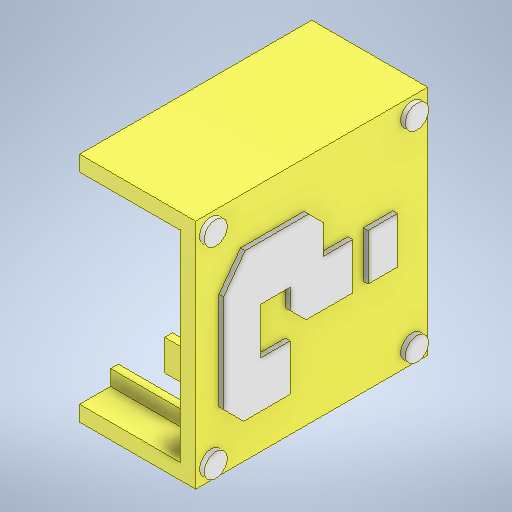
# Autodesk Inventor part: vraagblok2
Saved by Autodesk Inventor 2025 (Build 290162000, 162)
## iProperties
Created: 2024-05-27
Part Number: vraagblok2
Material: Generic
Document SubType Name: Modeling
Designer: wardv
Density: 1 g/cm^3
Appearance: Smooth - Yellow
Author: wardv
Autodesk Inventor part; units mm, degrees
ref_plane "YZ Plane" through (0, 0, 0) normal (1, 0, 0) x (0, 1, 0)
ref_plane "XZ Plane" through (0, 0, 0) normal (0, 1, 0) x (-1, 0, 0)
ref_plane "XY Plane" through (0, 0, 0) normal (0, 0, 1) x (1, 0, 0)
sketch "Sketch1" plane through (0, 0, 0) normal (0, 0, 1) x (1, 0, 0)
  line L0 (0, 0) -> (75, 0)
  line L1 (75, 0) -> (75, 150)
  line L2 (75, 150) -> (0, 150)
  line L3 (0, 150) -> (0, 0)
  dimension "d0" = 75
  dimension "d1" = 150
  constraints: 8 end point, 2 parallel, 1 horizontal, 1 perpendicular
  measures "d0" distance of L2.end L1.end
  measures "d1" distance between parallel lines of L0 L2
extrude "Extrusion1" add sketch "Sketch1" along normal blind 10
sketch "Sketch2" plane through (0, 0, 10) normal (0, 0, 1) x (1, 0, 0)
  line L0 (48, 85) -> (53, 85)
  line L1 (53, 85) -> (53, 19)
  line L2 (53, 19) -> (48, 19)
  line L3 (48, 19) -> (48, 14)
  line L4 (48, 14) -> (58, 14)
  line L5 (58, 14) -> (58, 90)
  line L6 (58, 90) -> (48, 90)
  line L7 (75, 150) -> (0, 150) projected
  line L8 (0, 150) -> (0, 0) projected
  line L9 (48, 85) -> (48, 90)
  dimension "d4" = 10
  dimension "d5" = 76
  dimension "d6" = 66
  dimension "d8" = 60
  dimension "d9" = 5
  dimension "d10" = 10
  dimension "d11" = 53
  dimension "d12" = 5
  dimension "d13" = 5
  constraints: 16 end point, 6 perpendicular, 1 horizontal
  measures "d4" distance of L5.end L6.end
  measures "d5" distance of L4.end L5.end
  measures "d6" distance of L0.end L1.end
  measures "d8" distance between parallel lines of L7 L6
  measures "d9" distance between parallel lines of L5 L1
  measures "d10" distance of L3.end L4.end
  measures "d11" distance between parallel lines of L8 L1
  measures "d12" distance of L2.end L3.end
  measures "d13" distance of L0.start L0.end
extrude "Extrusion2" add sketch "Sketch2" along normal blind 5
sketch "Sketch3" plane through (53, 19, 10) normal (-1, 0, 0) x (0, 0, 1)
  line L0 (5, 66) -> (5, 0) projected
  line L1 (5, 66) -> (3, 66)
  line L2 (3, 66) -> (3, 56)
  line L3 (3, 56) -> (5, 56)
  line L4 (5, 56) -> (5, 66)
  line L5 (5, 0) -> (5, -5) projected
  line L6 (5, 0) -> (3, 0)
  line L7 (3, 0) -> (3, 10)
  line L8 (3, 10) -> (5, 10)
  line L9 (5, 10) -> (5, 0)
  point P0 (-10, -19)
  point P1 (5, 10)
  point P2 (5, 56)
  dimension "d16" = 2
  dimension "d17" = 10
  dimension "d18" = 10
  dimension "d19" = 2
  constraints: 16 end point, 4 parallel, 2 horizontal, 2 perpendicular
  measures "d16" distance of L3.end L2.end
  measures "d17" distance of L1.end L2.end
  measures "d18" distance of L6.end L7.end
  measures "d19" distance between parallel lines of L0 L7
extrude "Extrusion3" add sketch "Sketch3" along normal blind 3
sketch "Sketch4" plane through (0, 0, 10) normal (0, 0, 1) x (1, 0, 0)
  line L0 (0, 150) -> (0, 0) projected
  line L1 (0, 10) -> (65, 10)
  line L2 (65, 10) -> (65, 140)
  line L3 (65, 140) -> (0, 140)
  line L4 (75, 150) -> (0, 150) projected
  line L5 (75, 0) -> (75, 150) projected
  line L6 (0, 0) -> (75, 0) projected
  point P0 (0, 140)
  dimension "d22" = 10
  dimension "d24" = 10
  dimension "d25" = 10
  constraints: 6 end point, 3 perpendicular, 1 point on line
  measures "d22" distance between parallel lines of L4 L3
  measures "d24" distance between parallel lines of L5 L2
  measures "d25" distance between parallel lines of L6 L1
extrude "Extrusion4" add sketch "Sketch4" along normal blind 140 contours L4 L5 L6 L0 L1 L2 L3
sketch "Sketch5" plane through (0, 10, 10) normal (0, 1, 0) x (1, 0, 0)
  line L0 (0, 10) -> (0, -140) projected
  line L1 (0, -115) -> (50, -115)
  line L2 (50, -115) -> (50, -85)
  line L3 (50, -85) -> (0, -85)
  line L4 (0, -115) -> (0, -120)
  line L5 (0, -120) -> (55, -120)
  line L6 (55, -120) -> (55, -80)
  line L7 (55, -80) -> (0, -80)
  line L8 (0, -85) -> (0, -80)
  line L9 (0, -140) -> (75, -140) projected
  dimension "d28" = 50
  dimension "d29" = 30
  dimension "d30" = 5
  dimension "d31" = 55
  dimension "d32" = 40
  dimension "d37" = 20
  constraints: 16 end point, 5 perpendicular, 4 point on line, 1 horizontal, 1 parallel
  measures "d28" distance of L1.start L1.end
  measures "d29" distance of L1.end L2.end
  measures "d30" distance of L1.start L4.end
  measures "d31" distance of L4.end L5.end
  measures "d32" distance of L5.end L6.end
  measures "d37" distance between parallel lines of L9 L5
extrude "Extrusion5" add sketch "Sketch5" along normal blind 10 contours L7 L6 L5 L0 L1 L2 L3
sketch "Sketch6" plane through (0, 10, 95) normal (0, 1, 0) x (1, 0, 0)
  line L0 (50, -30) -> (50, 0) projected
  line L1 (0, 0) -> (0, -30) projected
  line L2 (50, -30) -> (0, -30)
  line L3 (0, -30) -> (0, 0)
  line L4 (0, 0) -> (50, 0)
  line L5 (50, 0) -> (50, -30)
  point P0 (0, 95)
  point P1 (0, -30)
  constraints: 8 end point, 2 parallel, 1 horizontal, 1 perpendicular
extrude "Extrusion6" cut sketch "Sketch6" against normal blind 10
sketch "Sketch7" plane through (50, 0, 125) normal (-1, 0, 0) x (0, 0, 1)
  line L0 (-30, 0) -> (-30, 20) projected
  line L1 (0, 20) -> (0, 0) projected
  line L2 (-30, 20) -> (0, 20)
  line L3 (0, 20) -> (0, 17)
  line L4 (0, 17) -> (-30, 17)
  line L5 (-30, 17) -> (-30, 20)
  line L6 (0, 10) -> (-30, 10)
  line L7 (-30, 10) -> (-30, 13)
  line L8 (-30, 13) -> (0, 13)
  line L9 (0, 13) -> (0, 10)
  point P0 (-125, 0)
  point P1 (0, 13)
  point P2 (-30, 13)
  point P3 (0, 20)
  dimension "d38" = 3
  dimension "d39" = 3
  constraints: 16 end point, 4 parallel, 2 horizontal, 2 perpendicular, 2 point on line, 1 midpoint
  measures "d38" distance between parallel lines of L6 L8
  measures "d39" distance between parallel lines of L2 L4
extrude "Extrusion7" add sketch "Sketch7" along normal blind 5 contours L0 L8 L1 L6 | L0 L2 L1 L4
sketch "Sketch8" plane through (0, 0, 0) normal (-1, 0, 0) x (0, 0, 1)
  circle A0 centre (5, 120) radius 2.5
  circle A1 centre (5, 30) radius 2.5
  circle A2 centre (60, 5) radius 2.5
  circle A3 centre (120, 145) radius 2.5
  circle A4 centre (30, 145) radius 2.5
  line L0 (0, 0) -> (95, 0) projected
  line L1 (0, 150) -> (0, 0) projected
  line L2 (0, 150) -> (150, 150) projected
  line L3 (10, 140) -> (150, 140) projected
  line L4 (150, 150) -> (150, 140) projected
  dimension "d42" = 5
  dimension "d43" = 5
  dimension "d44" = 5
  dimension "d45" = 5
  dimension "d46" = 5
  dimension "d47" = 5
  dimension "d48" = 60
  dimension "d49" = 5
  dimension "d50" = 30
  dimension "d51" = 5
  dimension "d52" = 30
  dimension "d53" = 30
  dimension "d54" = 5
  dimension "d55" = 5
  dimension "d56" = 30
  constraints: 5 centre point
  measures "d42" diameter of A0
  measures "d43" diameter of A1
  measures "d44" diameter of A2
  measures "d45" diameter of A3
  measures "d46" diameter of A4
  measures "d47" distance from line of L0 A2.centre
  measures "d48" distance from line of L1 A2.centre
  measures "d49" distance from line of L1 A1.centre
  measures "d50" distance from line of L0 A1.centre
  measures "d51" distance from line of L1 A0.centre
  measures "d52" distance from line of L2 A0.centre
  measures "d53" distance from line of L1 A4.centre
  measures "d54" distance from line of L2 A4.centre
  measures "d55" distance from line of L3 A3.centre
  measures "d56" distance from line of L4 A3.centre
extrude "Extrusion8" cut sketch "Sketch8" against normal blind 5
sketch "Sketch9" plane through (75, 0, 0) normal (1, 0, 0) x (0, 0, -1)
  line L0 (-92, 25.5) -> (-92, 55.5)
  line L1 (-92, 55.5) -> (-111, 55.5)
  line L2 (-111, 55.5) -> (-111, 85.5)
  line L3 (-111, 85.5) -> (-92, 85.5)
  line L4 (-92, 85.5) -> (-92, 72.5)
  line L5 (-92, 72.5) -> (-81.582, 62.082)
  line L6 (-81.582, 62.082) -> (-51.582, 62.082)
  line L7 (-51.582, 62.082) -> (-51.582, 92.082)
  line L8 (-51.582, 92.082) -> (-70.582, 92.082)
  line L9 (-70.582, 92.082) -> (-70.582, 111.082)
  line L10 (-70.582, 111.082) -> (-80, 120.5)
  line L11 (-80, 120.5) -> (-121, 120.5)
  line L12 (-135, 38.5) -> (-122, 25.5)
  line L13 (-122, 25.5) -> (-92, 25.5)
  line L14 (-41.582, 62.082) -> (-22.582, 62.082)
  line L15 (-22.582, 62.082) -> (-22.582, 92.082)
  line L16 (-22.582, 92.082) -> (-41.582, 92.082)
  line L17 (-41.582, 92.082) -> (-41.582, 62.082)
  line L18 (-150, 0) -> (-150, 150) projected
  line L19 (0, 150) -> (-150, 150) projected
  line L20 (-135, 38.5) -> (-135, 101.5)
  line L21 (-135, 101.5) -> (-121, 120.5)
  line L22 (-10, 10) -> (-150, 10) projected
  circle A0 centre (-140, 10) radius 7.5
  line L23 (-10, 140) -> (-150, 140) projected
  circle A1 centre (-140, 140) radius 7.5
  line L24 (-10, 10) -> (-90, 10) projected
  circle A2 centre (-10, 10) radius 7.5
  line L25 (-10, 140) -> (-10, 10) projected
  circle A3 centre (-10, 140) radius 7.5
  line L26 (0, 0) -> (0, 150) projected
  point P0 (-100.5, 120.5)
  point P1 (-51.582, 77.082)
  point P2 (-135, 70)
  dimension "d59" = 30
  dimension "d60" = 19
  dimension "d61" = 30
  dimension "d62" = 19
  dimension "d63" = 13
  dimension "d64" = 30
  dimension "d65" = 30
  dimension "d66" = 19
  dimension "d67" = 19
  dimension "d68" = 41
  dimension "d69" = 30
  dimension "d76" = 13
  dimension "d80" = 19
  dimension "d81" = 10
  dimension "d85" = 95
  dimension "d86" = 63
  dimension "d87" = 80
  dimension "d88" = 15
  dimension "d89" = 15
  dimension "d90" = 15
  dimension "d91" = 15
  dimension "d92" = 15
  dimension "d93" = 10
  dimension "d94" = 10
  dimension "d95" = 10
  constraints: 40 end point, 8 perpendicular, 6 parallel, 4 centre point, 3 midpoint, 3 point on line, 3 vertical, 1 coincident, 1 horizontal
  measures "d59" distance of L0.start L0.end
  measures "d60" distance of L0.end L1.end
  measures "d61" distance of L1.end L2.end
  measures "d62" distance of L2.end L3.end
  measures "d63" distance of L3.end L4.end
  measures "d64" distance of L5.end L6.end
  measures "d65" distance of L6.end L7.end
  measures "d66" distance of L7.end L8.end
  measures "d67" distance of L8.end L9.end
  measures "d68" distance of L10.end L11.end
  measures "d69" distance of L12.end L0.start
  measures "d76" horizontal distance of L12.end L12.start
  measures "d80" distance of L16.end L15.end
  measures "d81" distance from line of L17 point (-51.582, 77.082)
  measures "d85" vertical distance of L11.end L12.end
  measures "d86" distance of L12.start L20.end
  measures "d87" distance from line of L19 point (-135, 70)
  measures "d88" distance between parallel lines of L18 L20
  measures "d89" diameter of A0
  measures "d90" diameter of A1
  measures "d91" diameter of A2
  measures "d92" diameter of A3
  measures "d93" distance from line of L18 A0.centre
  measures "d94" distance from line of L26 A2.centre
  measures "d95" distance from line of L18 A1.centre
extrude "Extrusion9" add sketch "Sketch9" along normal blind 3 contours L13 L12 L20 L21 L11 L10 L9 L8 L7 L6 L5 L4 L3 L2 L1 L0 | L17 L16 L15 L14 | A0 L22 | L22 A0 | A1 L23 | L23 A1 | A3 L25 L23 | L23 L25 A3 | A2 L25 L22 | L22 L25 A2
body "Solid1"
